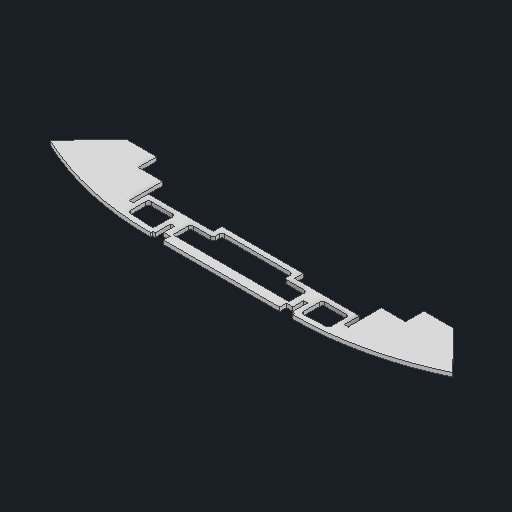
# Autodesk Inventor part: main
Saved by Autodesk Inventor 2024 (Build 280153000, 153)
## iProperties
Created: 2022-03-21
Part Number: main
Material: Generic
Document SubType Name: Modeling
Designer: kardo
Density: 1 g/cm^3
Appearance: Default
Mass: 20.1247 g
Surface Area: 169.415 cm^2
Volume: 20.1247 cm^3
Author: kardo
Autodesk Inventor part; units mm, degrees
ref_plane "YZ Plane" through (0, 0, 0) normal (1, 0, 0) x (0, 1, 0)
ref_plane "XZ Plane" through (0, 0, 0) normal (0, 1, 0) x (-1, 0, 0)
ref_plane "XY Plane" through (0, 0, 0) normal (0, 0, 1) x (1, 0, 0)
derived "parameters_frame.ipt"
derived "stencil_frame.ipt"
sketch "sk_joint_locations" plane through (81.12, 0, 0) normal (1, 0, 0) x (0, 1, 0)
  line L0 (0, 0) -> (122.4, 9.6331) construction
  line L1 (36.465, 28.832) -> (112.2, 28.832) construction
  arc A0 (36.465, 28.832) -> (11.22, 28.376) centre (36.465, -670.197) ccw construction
  line L2 (-241.5001, 19.2432) -> (11.22, 28.376) construction
  line L3 (-345, 16.32) -> (-262.2001, 18.586) construction
  arc A1 (-262.2001, 18.586) -> (-241.5001, 19.2432) centre (-326.8578, 2381.2399) ccw construction
  line L4 (-122.4795, 3121.122) -> (270.8781, -1876.9598) construction
  line L5 (-230.0001, 3089.1136) -> (-230.0001, -1866.0023) construction
  line L6 (-114.9999, 3089.1136) -> (-114.9999, -1866.0023) construction
  line L7 (-345, 3089.1136) -> (-345, -1866.0023) construction
  line L8 (0, 3089.1136) -> (0, -1866.0023) construction
  line L9 (529.622, 47.2379) -> (-602.608, 2.7525) construction
  line L10 (-673.1615, -36.5999) -> (647.9226, 67.3717) construction
  line L11 (189.4528, 29.5173) -> (189.1111, 38.2146) construction
  line L12 (201.105, 36.5853) -> (201.7901, 27.8813) construction
  line L13 (0, 14.144) -> (121.9006, 15.9783) construction
  line L14 (-230.0001, 45.8224) -> (-230.0001, 19.6588) construction
  line L15 (-345, 37.3935) -> (-345, 16.32) construction
  line L16 (-114.9999, 50.9907) -> (-114.9999, 23.8147) construction
  line L17 (0, 52.89) -> (0, 27.9705) construction
  line L18 (119.1768, 50.5875) -> (119.7216, 43.6656) construction
  line L19 (120.2663, 36.7438) -> (119.7216, 43.6656) construction
  line L20 (120.2663, 36.7438) -> (120.8111, 29.822) construction
  line L21 (120.8111, 29.822) -> (121.3559, 22.9001) construction
  line L22 (121.3559, 22.9001) -> (121.9006, 15.9783) construction
  line L23 (0, 14.144) -> (0, 0) construction
  spline S0 degree 4 poles (-345, 37.3935) (-258.8686, 45.1235) (-172.5923, 49.7074) (-86.3167, 52.89) (0, 52.89) knots 0 0 0 0 0 1 1 1 1 1
  spline S1 degree 3 poles (0, 52.89) (92.8353, 52.89) (195.0311, 49.5089) (255, 36.448) knots 0 0 0 0 1 1 1 1
  spline S2 degree 2 poles (122.4, 9.6331) (190.08, 14.9596) (255, 36.448) knots 0 0 0 1 1 1
  line L24 (112.2, 37.536) -> (112.2, 28.832) construction
  line L25 (112.2, 35.848) -> (112.2, 30.52) construction
  point P0 (-122.4795, 3121.122)
  point P1 (270.8781, -1876.9598)
  point P2 (189.282, 33.8659)
  point P3 (201.4475, 32.2333)
  point P4 (134.9575, 11.3411)
  point P5 (-345, 26.8568)
  point P6 (-230.0001, 32.7406)
  point P7 (-114.9999, 37.4027)
  point P8 (0, 40.4303)
  point P9 (112.2, 33.184)
sketch "sk_cowl_joint_locations" plane through (54.6, 0, 0) normal (1, 0, 0) x (0, 1, 0)
  line L0 (-345, 16.32) -> (-262.2001, 18.586) construction
  arc A0 (-262.2001, 18.586) -> (-241.5001, 19.2432) centre (-326.8578, 2381.2399) ccw construction
  line L1 (-241.5001, 19.2432) -> (11.22, 28.376) construction
  arc A1 (36.465, 28.832) -> (11.22, 28.376) centre (36.465, -670.197) ccw construction
  line L2 (36.465, 28.832) -> (112.2, 28.832) construction
  line L3 (94.8, 29.632) -> (36.465, 29.632) construction
  arc A2 (36.465, 29.632) -> (11.1911, 29.1755) centre (36.465, -670.197) ccw construction
  line L4 (11.1911, 29.1755) -> (-241.529, 20.0427) construction
  arc A3 (-262.222, 19.3857) -> (-241.529, 20.0427) centre (-326.8578, 2381.2399) ccw construction
  line L5 (-262.222, 19.3857) -> (-345, 17.1203) construction
  line L6 (-230.0001, 3089.1136) -> (-230.0001, -1866.0023) construction
  line L7 (-114.9999, 3089.1136) -> (-114.9999, -1866.0023) construction
  line L8 (-345, 3089.1136) -> (-345, -1866.0023) construction
  line L9 (0, 3089.1136) -> (0, -1866.0023) construction
  line L10 (-230.0001, 44.8681) -> (-230.0001, 20.4593) construction
  line L11 (-114.9999, 49.7658) -> (-114.9999, 24.6152) construction
  line L12 (-345, 17.1203) -> (-345, 17.1203)
  line L13 (-345, 17.1203) -> (-345, 36.7228) construction
  line L14 (-850.7464, 3011.9134) -> (325.2296, -1886.3794) construction
  line L15 (-344.7454, 36.7228) -> (-345, 39.712) construction
  line L16 (0, 51.4) -> (0, 28.7711) construction
  spline S0 degree 2 poles (-345, 39.712) (-172.656, 54.3934) (0, 54.4) knots 0 0 0 1 1 1
  spline S1 degree 3 poles (0, 54.4) (37.026, 54.4) (80.784, 47.9917) (112.2, 37.536) knots 1 1 1 1 2 2 2 2
  spline S2 degree 3 poles (111.2526, 34.6895) (106.0906, 36.4075) (96.4401, 39.2282) (84.5011, 42.0313) (75.2591, 43.9395) (68.9709, 45.1125) (60.9945, 46.449) (54.5373, 47.4124) (46.413, 48.4791) (39.8882, 49.2203) (31.7426, 50.0013) (25.2514, 50.5076) (17.2112, 50.9875) (9.2661, 51.3118) (3.0567, 51.4) (0, 51.4) knots 1 1 1 1 1.166667 1.291667 1.333333 1.416667 1.458333 1.541667 1.583333 1.666667 1.708333 1.791667 1.833333 1.916667 2 2 2 2
  spline S3 degree 3 poles (0, 51.4) (-19.1698, 51.3993) (-52.712, 51.1604) (-91.0357, 50.4121) (-119.7742, 49.6473) (-138.931, 49.0355) (-162.8744, 48.1436) (-182.0269, 47.3282) (-205.9648, 46.1816) (-225.113, 45.1626) (-249.0455, 43.7615) (-268.1894, 42.5387) (-292.1166, 40.883) (-316.041, 39.1) (-335.1777, 37.5379) (-344.7454, 36.7228) knots 0 0 0 0 0.166667 0.291667 0.333333 0.416667 0.458333 0.541666 0.583333 0.666666 0.708333 0.791666 0.833333 0.916666 1 1 1 1
  line L17 (-144.5331, 44.6212) -> (-139.5174, 23.7292) construction
  line L18 (-134.9371, 30.3529) -> (-140.7713, 28.9522) construction
  line L19 (-137.4449, 40.7989) -> (-143.2792, 39.3982) construction
  line L20 (-144.5331, 44.6212) -> (-138.6989, 46.0219) construction
  line L21 (-139.5174, 23.7292) -> (-133.6831, 25.1299) construction
  line L22 (-138.6989, 46.0219) -> (-138.9044, 52.0184) construction
  point P0 (0, 0)
  point P1 (-345, 26.9216)
  point P2 (-230.0001, 32.6637)
  point P3 (-114.9999, 37.1905)
  point P4 (0, 40.0855)
  point P5 (-850.7464, 3011.9134)
  point P6 (325.2296, -1886.3794)
  point P7 (-85.2629, 50.788)
  point P8 (0, 40.0855)
sketch "sk_main_base" plane through (0, 0, 0) normal (0, 1, 0) x (-1, 0, 0)
  line L0 (0, -1866.0023) -> (0, 3089.1136) construction
  line L1 (-81.12, 14.144) -> (-107.2232, 45.2526) construction
  spline S0 degree 2 poles (-54.6, 54.4) (-107.2974, 54.4) (-156, 31.008) knots 0 0 0 1 1 1 construction
  line L2 (0, 54.4) -> (-54.6, 54.4) construction
  line L3 (0, 22.1303) -> (-31.32, 22.1303)
  line L4 (-31.32, 22.1303) -> (-31.32, 28.7705)
  line L5 (-31.32, 28.7705) -> (-81.12, 28.7705)
  line L6 (-81.12, 40.4303) -> (-81.12, 28.7705)
  line L7 (-81.12, 40.4303) -> (-84.12, 40.4303)
  line L8 (-84.12, 40.4303) -> (-84.12, 14.944)
  line L9 (-125.7085, 0.8) -> (-154.6529, 30.7649)
  line L10 (-54.6, 53.6) -> (0, 53.6)
  line L11 (0, 53.6) -> (0, 22.1303)
  line L12 (-156, 31.008) -> (-126.048, 0) construction
  line L13 (-126.048, 0) -> (-81.12, 0) construction
  line L14 (-84.12, 14.944) -> (-102.6854, 14.944)
  line L15 (-102.6854, 14.944) -> (-102.6854, 0.8)
  line L16 (-102.6854, 0.8) -> (-125.7085, 0.8)
  line L17 (-102.6854, 14.144) -> (-102.6854, 0) construction
  spline S1 degree 5 poles (-155.6536, 30.2869) (-136.7957, 39.3429) (-117.0148, 46.4727) (-96.4408, 51.2945) (-75.5189, 53.5986) (-54.6, 53.6) knots 0 0 0 0 0 0 1 1 1 1 1 1
  point P0 (0, 0)
  point P1 (-34.32, 21.3303)
  point P2 (-34.32, 27.9705)
  dimension "d3" = 0.8
  dimension "d5" = 3
  dimension "d6" = 0.8
  dimension "d7" = 0.8
  dimension "d8" = 3
  dimension "d11" = 0.8
  dimension "d12" = 0.8
  dimension "d13" = 0.8
  constraints: 24 end point, 6 parallel, 4 perpendicular, 2 collinear, 1 point on line, 4 other
  measures "d5" distance of L6.start L7.end
  measures "d6" distance from line of point (-34.32, 27.971) L5
  measures "d7" distance from line of L3 point (-34.32, 21.33)
  measures "d8" distance from line of L4 point (-34.32, 27.971)
  measures "d11" distance from line of L1.start L14
  measures "d12" distance between parallel lines of L13 L16
  measures "d13" distance between parallel lines of L12 L9
extrude "thicken" add sketch "sk_main_base" along normal blind 3
sketch "sk_stringer_cowl_cut" plane through (0, 0, 0) normal (0, 1, 0) x (-1, 0, 0)
  line L0 (-54.6, -1866.0023) -> (-54.6, 3089.1136) construction
  line L1 (-49.6, 90.0855) -> (-52.6, 90.0855)
  line L2 (-52.6, 90.0855) -> (-52.6, 40.0855)
  line L3 (-52.6, 40.0855) -> (-49.6, 40.0855)
  line L4 (-49.6, 40.0855) -> (-49.6, 90.0855)
  point P0 (0, 0)
  point P1 (-54.6, 40.0855)
  dimension "d14" = 5
  dimension "d15" = 3
  dimension "d20" = 50
  constraints: 8 end point, 3 parallel, 1 horizontal, 1 perpendicular, 1 point on line
  measures "d14" distance between parallel lines of L0 L4
  measures "d15" distance between parallel lines of L4 L2
  measures "d20" distance of L3.end L1.start
extrude "cut_joint" cut sketch "sk_stringer_cowl_cut" along normal through all both and the other way through all
sketch "sk_cowl_liner_cut" plane through (0, 0, 0) normal (0, 1, 0) x (-1, 0, 0)
  line L0 (0, 54.4) -> (-54.6, 54.4) projected
  line L1 (-54.6, 54.4) -> (-54.6, 52.1)
  line L2 (-54.6, 52.1) -> (-49.6, 52.1)
  line L3 (-49.6, 52.1) -> (-49.6, 48.4)
  line L4 (-49.6, 48.4) -> (-44.6, 48.4)
  line L5 (-44.6, 48.4) -> (-44.6, 54.4)
  point P0 (0, 0)
  dimension "d21" = 2.3
  dimension "d23" = 5
  dimension "d24" = 5
  dimension "d40" = 6
  constraints: 10 end point, 3 perpendicular, 2 parallel, 1 point on line
  measures "d21" distance between parallel lines of L0 L2
  measures "d23" distance of L1.end L2.end
  measures "d24" distance of L3.end L4.end
  measures "d40" distance of L4.end L5.end
extrude "cut_liner" cut sketch "sk_cowl_liner_cut" along normal through all both and the other way through all
sketch "sk_cut_weight" plane through (0, 0, 0) normal (0, 1, 0) x (-1, 0, 0)
  line L0 (0, 22.1303) -> (-31.32, 22.1303) construction
  line L1 (-31.32, 22.1303) -> (-31.32, 28.7705) construction
  line L2 (-31.32, 28.7705) -> (-81.12, 28.7705) construction
  line L3 (-81.12, 40.4303) -> (-81.12, 28.7705) construction
  spline S0 degree 3 poles (-155.6536, 30.2869) (-152.9564, 31.5824) (-147.5437, 34.0653) (-140.7324, 36.8988) (-133.8869, 39.5297) (-128.3831, 41.4725) (-121.4692, 43.6985) (-115.9106, 45.3173) (-108.928, 47.1385) (-103.3144, 48.4335) (-96.2629, 49.8499) (-90.5941, 50.8211) (-83.4735, 51.8328) (-77.7493, 52.4803) (-70.5594, 53.0874) (-63.3347, 53.4921) (-57.5178, 53.6) (-54.6, 53.6) knots 0 0 0 0 0.083333 0.166667 0.208333 0.291667 0.333333 0.416667 0.458333 0.541667 0.583333 0.666667 0.708333 0.791667 0.833333 0.916667 1 1 1 1 construction
  line L4 (-44.6, 48.4) -> (-44.6, 54.4) construction
  line L5 (-49.6, 48.4) -> (-44.6, 48.4) construction
  line L6 (-49.6, 52.1) -> (-49.6, 48.4) construction
  line L7 (0, -1866.0023) -> (0, 3089.1136) projected
  line L8 (0, 26.1303) -> (-27.32, 26.1303)
  line L9 (-27.32, 26.1303) -> (-27.32, 32.7705)
  line L10 (-27.32, 32.7705) -> (-44.6, 32.7705)
  line L11 (-44.6, 32.7705) -> (-44.6, 46.4)
  line L12 (-44.6, 46.4) -> (0, 46.4)
  line L13 (-56.6, 49.6) -> (-56.6, 32.7705)
  line L14 (-56.6, 32.7705) -> (-77.12, 32.7705)
  line L15 (-77.12, 32.7705) -> (-77.12, 48.5106)
  line L16 (-77.12, 48.5106) -> (-56.6, 49.6)
  line L17 (-49.6, 28.7705) -> (-49.6, 48.4) construction
  line L18 (-52.6, 28.7705) -> (-52.6, 48.4) construction
  line L19 (-52.6, 48.4) -> (-49.6, 48.4) construction
  line L20 (-77.12, 48.5106) -> (-77.12, 52.5106) construction
  point P0 (0, 0)
  dimension "d27" = 3
  dimension "d28" = 4
  dimension "d29" = 4
  dimension "d30" = 4
  dimension "d31" = 4
  dimension "d32" = 4
  dimension "d33" = 4
  dimension "d34" = 4
  dimension "d35" = 4
  dimension "d36" = 2
  constraints: 26 end point, 9 parallel, 4 point on line, 3 collinear, 1 perpendicular, 1 other
  measures "d27" distance between parallel lines of L17 L18
  measures "d28" distance between parallel lines of L18 L13
  measures "d29" distance between parallel lines of L2 L14
  measures "d30" distance between parallel lines of L3 L15
  measures "d31" distance of L15.end L20.end
  measures "d32" vertical distance of point (-54.6, 53.6) L13.start
  measures "d33" distance between parallel lines of L2 L10
  measures "d34" distance between parallel lines of L1 L9
  measures "d35" distance between parallel lines of L0 L8
  measures "d36" distance between parallel lines of L12 L5
extrude "cut_weight" cut sketch "sk_cut_weight" along normal through all both and the other way through all
fillet "rounding" radius 2 7 edges at (77.12, 1.5, 32.7705) (27.32, 1.5, 26.1303) (27.32, 1.5, 32.7705) (44.6, 1.5, 32.7705) (77.12, 1.5, 48.5106) (56.6, 1.5, 49.6) (56.6, 1.5, 32.7705)
mirror "mirror" about plane through (0, 0, 0) normal (1, 0, 0)
equation "\"d3\" = shell_thickness"
equation "\"d5\" = stringer_thickness"
equation "\"d6\" = shell_thickness"
equation "\"d7\" = shell_thickness"
equation "\"d8\" = bulkhead_thickness"
equation "\"d11\" = shell_thickness"
equation "\"d12\" = shell_thickness"
equation "\"d13\" = shell_thickness"
equation "\"d9\" = bulkhead_thickness"
equation "\"d14\" = cowl_liner_width"
equation "\"d15\" = bulkhead_thickness"
equation "\"d21\" = cowl_liner_thickness + shell_thickness"
equation "\"d23\" = cowl_liner_width"
equation "\"d24\" = cowl_sealing_width"
equation "\"d40\" = cowl_sealing_thickness + cowl_shell_thickness + cowl_liner_thickness"
equation "\"d27\" = bulkhead_thickness"
equation "\"d28\" = bulkhead_inset"
equation "\"d29\" = bulkhead_inset"
equation "\"d30\" = bulkhead_inset"
equation "\"d31\" = bulkhead_inset"
equation "\"d32\" = bulkhead_inset"
equation "\"d33\" = bulkhead_inset"
equation "\"d34\" = bulkhead_inset"
equation "\"d35\" = bulkhead_inset"
equation "\"shell_thickness\" = 0.8"
equation "\"stringer_thickness\" = 3"
equation "\"bulkhead_thickness\" = 3"
equation "\"cowl_liner_width\" = 5"
equation "\"cowl_liner_thickness\" = 1.5"
equation "\"cowl_sealing_width\" = 5"
equation "\"cowl_sealing_thickness\" = 3"
equation "\"cowl_shell_thickness\" = 1.5"
equation "\"bulkhead_inset\" = 4"
body "Solid1"
